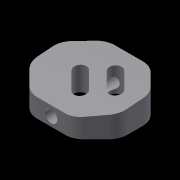
# Autodesk Inventor part: PinkyRouter
Saved by Autodesk Inventor 2015 (Build 190159000, 159)
## iProperties
Created: 2014-11-12
Part Number: PinkyRouter
Material: Generic
Document SubType Name: Modeling
Designer: Inventor
Density: 1 g/cm^3
Appearance: Default
Mass: 0.451381 g
Surface Area: 5.61533 cm^2
Volume: 0.451381 cm^3
Author: Inventor
Autodesk Inventor part; units mm, degrees
ref_plane "YZ Plane" through (0, 0, 0) normal (1, 0, 0) x (0, 1, 0)
ref_plane "XZ Plane" through (0, 0, 0) normal (0, 1, 0) x (-1, 0, 0)
ref_plane "XY Plane" through (0, 0, 0) normal (0, 0, 1) x (1, 0, 0)
sketch "Base" plane through (0, 0, 0) normal (0, 0, 1) x (1, 0, 0)
  line L0 (-7.25, -2.5) -> (-7.25, 2.5)
  line L1 (-7.25, 2.5) -> (-3.5, 6.25)
  line L2 (-3.5, 6.25) -> (3.5, 6.25)
  line L3 (3.5, 6.25) -> (7.25, 2.5)
  line L4 (7.25, 2.5) -> (7.25, -2.5)
  line L5 (7.25, -2.5) -> (3.5, -6.25)
  line L6 (3.5, -6.25) -> (-3.5, -6.25)
  line L7 (-3.5, -6.25) -> (-7.25, -2.5)
  line L8 (-7.25, 0) -> (7.25, 0) construction
  line L9 (0, 6.25) -> (0, -6.25) construction
  point P0 (0, 0)
  point P1 (0, 0)
  dimension "d1" = 14.5
  dimension "d5" = 12.5
  dimension "d7" = 5
  constraints: 20 end point, 7 midpoint, 4 parallel, 3 perpendicular, 2 vertical, 1 coincident, 1 horizontal
  measures "d1" distance between parallel lines of L4 L0
  measures "d5" distance between parallel lines of L6 L2
  measures "d7" distance of L3.end L4.end
extrude "BaseFeature" add sketch "Base" along normal blind 4
fillet "BaseFilletsFeature" radius 3 8 edges at (-7.25, -2.5, 2) (-3.5, -6.25, 2) (3.5, -6.25, 2) (7.25, -2.5, 2) (7.25, 2.5, 2) (3.5, 6.25, 2) (-3.5, 6.25, 2) (-7.25, 2.5, 2)
sketch "RailHoles" plane through (0, 0, 4) normal (0, 0, 1) x (1, 0, 0)
  line L0 (1.2713, 2.8219) -> (3.8219, 0.2713) construction
  line L1 (-1.7718, 0.2081) -> (0.7788, -2.3425) construction
  line L2 (6.3713, 3.3787) -> (4.3787, 5.3713) construction
  line L3 (5.375, 4.375) -> (2.5466, 1.5466) construction
  circle A0 centre (1.2713, 2.8219) radius 1
  circle A1 centre (3.8219, 0.2713) radius 1
  circle A2 centre (-1.7718, 0.2081) radius 1
  circle A3 centre (0.7788, -2.3425) radius 1
  line L4 (1.9784, 3.529) -> (4.529, 0.9784)
  line L5 (0.5642, 2.1148) -> (3.1148, -0.4358)
  line L6 (-1.0647, 0.9152) -> (1.4859, -1.6354)
  line L7 (-2.4789, -0.499) -> (0.0717, -3.0496)
  dimension "d11" = 4
  dimension "d12" = 4
  dimension "d13" = 3.6071
  dimension "d14" = 2
  dimension "d15" = 1.5
  dimension "d25" = 2.818
  constraints: 14 end point, 8 point on circle, 8 tangent, 4 centre point, 4 coincident, 3 equal radius, 3 parallel, 2 midpoint, 1 perpendicular
  measures "d11" distance between parallel lines of L2 L0
  measures "d12" distance between parallel lines of L0 L1
  measures "d13" distance of L0.start L0.end
  measures "d14" diameter of A0
  measures "d15" distance from line of L1.end L3
  measures "d25" distance of L2.start L2.end
extrude "RailHolesFeature" cut sketch "RailHoles" against normal through all
sketch "RouteHole" plane through (-2.2574, -6.25, 0) normal (0, -1, 0) x (1, 0, 0)
  line L0 (4.5147, 4) -> (4.5147, 0) construction
  line L1 (0, 4) -> (4.5147, 4) construction
  line L2 (0, 0) -> (0, 4) construction
  line L3 (4.5147, 0) -> (0, 0) construction
  line L4 (0, 4) -> (0, 0) construction
  line L5 (0, 4) -> (4.5147, 4) construction
  line L6 (2.2574, 4) -> (2.2574, 0) construction
  line L7 (4.5147, 0) -> (0, 0) construction
  circle A0 centre (2.2574, 1.5) radius 1.25
  dimension "d40" = 2.5
  dimension "d41" = 1.5
  constraints: 2 end point, 2 midpoint, 1 centre point, 1 point on line
  measures "d40" diameter of A0
  measures "d41" distance from line of L3 A0.centre
hole "RouteHoleFeature" at (0, -6.25, 1.5) direction (0, 1, 0) diameter 2 end through all
sketch "SideProfile" plane through (7.25, -1.2574, 0) normal (1, 0, 0) x (0, 0, -1)
  arc A0 (-4, 7.5074) -> (-3, -4.9926) centre (74.625, 7.5074) ccw
  line L0 (-4, -4.9926) -> (0, -4.9926) construction
  line L1 (0, 7.5074) -> (-4, 7.5074) construction
  line L2 (-3, -4.9926) -> (0, -4.9926)
  line L3 (0, 7.5074) -> (0, -4.9926)
  line L4 (0, 7.5074) -> (0, 6.6287) projected
  line L5 (0, 7.5074) -> (-4, 7.5074)
  line L6 (-4, -2.1213) -> (-4, 0) construction
  dimension "d36" = 4
  dimension "d39" = 3
  constraints: 6 end point, 2 collinear, 2 point on circle, 2 point on line, 1 centre point, 1 perpendicular, 1 tangent
  measures "d36" distance of L1.start L5.end
  measures "d39" distance of L0.end L2.start
extrude "SideProfileFeature" cut sketch "SideProfile" against normal through all keep common part
equation "\"d7\" = 0.4 * d5"
equation "\"d12\" = 2 * d14"
equation "\"d13\" = 1.28 * d25"
